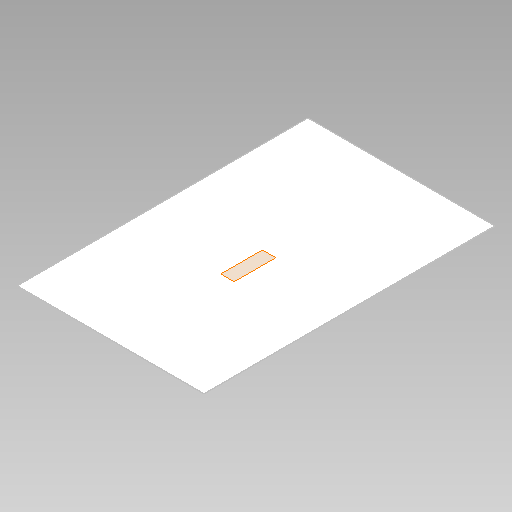
# Autodesk Inventor part: ground
Saved by Autodesk Inventor 2021 (Build 250183000, 183)
## iProperties
Created: 2020-05-21
Part Number: ground
Material: Generic
Document SubType Name: Modeling
Designer: Hannah
Density: 1 g/cm^3
Appearance: Gray
Mass: 3.27631e+06 g
Surface Area: 2.63278e+06 cm^2
Volume: 3.27631e+06 cm^3
Author: Hannah
Autodesk Inventor part; units mm, degrees
ref_plane "YZ Plane" through (0, 0, 0) normal (1, 0, 0) x (0, 1, 0)
ref_plane "XZ Plane" through (0, 0, 0) normal (0, 1, 0) x (-1, 0, 0)
ref_plane "XY Plane" through (0, 0, 0) normal (0, 0, 1) x (1, 0, 0)
ref_plane "Work Plane1" through (0, -310, 0) normal (0, 1, 0) x (-1, 0, 0)
sketch "Sketch1" plane through (0, -310, 0) normal (0, 1, 0) x (-1, 0, 0)
  line L0 (4830.0712, 6592.7226) -> (-4346.7416, 6592.7226)
  line L1 (-4346.7416, 6592.7226) -> (-4346.7416, -7688.0921)
  line L2 (-4346.7416, -7688.0921) -> (4830.0712, -7688.0921)
  line L3 (4830.0712, -7688.0921) -> (4830.0712, 6592.7226)
  point P0 (0, 0)
  constraints: 8 end point, 2 parallel, 1 horizontal, 1 perpendicular
extrude "Extrusion1" add sketch "Sketch1" against normal blind 25
body "Solid1"
